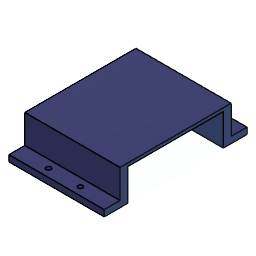
CubrePilas (Autodesk Fusion 360 design; units mm, degrees)
Autodesk Fusion 360 part; units mm, degrees
note: some values were not read from the file. Set by a fixed rule: which sketch regions a step uses.
sketch "Boceto2" plane through (0, 4, 0) normal (0, 1, 0) x (-1, 0, 0)
  line L0 (9, 0) -> (-1, 0)
  line L1 (-30, 0) -> (-60, 0)
  line L2 (-30, 0) -> (0, 0)
  line L3 (-30, 25) -> (-30, -10)
  line L4 (-30, -10) -> (-60, -10)
  line L5 (-60, -10) -> (-60, 60)
  line L6 (-60, 60) -> (0, 60)
  line L7 (0, 60) -> (0, -10)
  line L8 (0, -10) -> (-30, -10)
  line L9 (0, -10) -> (-5, -10)
  line L10 (-5, -10) -> (-5, -5)
  line L11 (-5, -5) -> (-55, -5)
  line L12 (-55, -5) -> (-55, 55)
  line L13 (-55, 55) -> (-5, 55)
  line L14 (-5, 55) -> (-5, -5)
  dimension "d1" = 10
  dimension "d2" = 30
  dimension "d3" = 30
  dimension "d4" = 35
  dimension "d5" = 70
  dimension "d6" = 5
  dimension "d7" = 5
  dimension "d8" = 50
  dimension "d9" = 60
  constraint horizontal L0
  constraint horizontal L1
  constraint parallel L1 L2
  constraint perpendicular L2 L3
  constraint perpendicular L3 L4
  constraint perpendicular L1 L5
  constraint perpendicular L3 L6
  constraint perpendicular L4 L7
  constraint perpendicular L3 L8
  constraint perpendicular L7 L9
  constraint perpendicular L9 L10
  constraint perpendicular L5 L11
  constraint perpendicular L1 L12
  constraint perpendicular L12 L13
  constraint perpendicular L11 L14
  measures "d1" distance of L0.start L0.end
  measures "d2" distance of L1.start L1.end
  measures "d3" distance of L1.start L2.end
  measures "d4" distance of L3.start L3.end
  measures "d5" distance of L4.end L5.end
  measures "d6" distance of L7.end L9.end
  measures "d7" distance of L9.end L10.end
  measures "d8" distance of L10.end L11.end
  measures "d9" distance of L11.end L12.end
extrude "Extruir1" add sketch "Boceto2" along normal blind 20 contours L0 L2 L7 L8 L9 L10 L14 | L0 L1 L2 L5 L6 L7 L12 L13 L14 | L3 L8 L10 L11 | L1 L3 L4 L5 L11 L12
sketch "Boceto3" plane through (0, 4, 0) normal (0, 1, 0) x (-1, 0, 0)
  line L0 (0, -10) -> (-5, -10)
  line L1 (-5, -10) -> (-10, -20)
  line L2 (0, -10) -> (0, -20)
  line L3 (0, -20) -> (-60, -20)
  line L4 (-60, -20) -> (-60, -10)
  line L5 (-60, -10) -> (-64.5056, 6.5239)
  line L6 (0, 60) -> (0, 70)
  line L7 (0, 70) -> (-60, 70)
  line L8 (-60, 70) -> (-60, 60)
  line L9 (-60, 60) -> (0, 60)
  line L10 (-5, -10) -> (-60, -10)
  dimension "d12" = 10
  dimension "d13" = 10
  constraint horizontal L0
  constraint perpendicular L0 L2
  constraint perpendicular L2 L3
  constraint perpendicular L3 L4
  constraint vertical L6
  constraint perpendicular L6 L7
  constraint perpendicular L7 L8
  constraint perpendicular L6 L9
  constraint perpendicular L4 L10
  measures "d12" distance of L0.start L2.end
  measures "d13" distance of L6.start L6.end
extrude "Extruir2" add sketch "Boceto3" along normal blind 4
sketch "Boceto4" plane through (0, 8, 0) normal (0, 1, 0) x (-1, 0, 0)
  line L0 (0, -10) -> (-60, -10)
  line L1 (-60, -10) -> (-60, -20)
  line L2 (-60, -20) -> (0, -20)
  line L3 (0, -20) -> (0, -10)
  line L4 (0, -15) -> (-20, -15)
  line L5 (-26, -15) -> (-35, -15)
  line L6 (-20, -15) -> (-40, -15)
  line L7 (-40, -15) -> (-80, 70)
  line L8 (0, 70) -> (0, 65)
  line L9 (0, 65) -> (-20, 65)
  line L10 (-20, 65) -> (-40, 65)
  circle A0 centre (-40, 65) radius 1.5
  circle A1 centre (-20, 65) radius 1.5
  circle A2 centre (-20, -15) radius 1.5
  circle A3 centre (-40, -15) radius 1.5
  dimension "d16" = 20
  dimension "d17" = 3
  dimension "d18" = 3
  dimension "d19" = 3
  dimension "d20" = 3
  constraint midpoint L3 L4.start
  constraint perpendicular L1 L4
  constraint parallel L4 L5
  constraint parallel L5 L6
  constraint vertical L8
  constraint perpendicular L8 L9
  constraint perpendicular L8 L10
  constraint coincident L10.end A0.centre
  constraint coincident L9.end L10.start
  constraint coincident L4.end L6.start
  constraint coincident L6.end L7.start
  measures "d16" distance of L4.start L4.end
  measures "d17" diameter of A0
  measures "d18" diameter of A1
  measures "d19" diameter of A2
  measures "d20" diameter of A3
extrude "Extruir3" cut sketch "Boceto4" against normal blind 30 contours L6 L7 A3 | L6 L7 A3 | L4 L6 A2 | L4 L6 A2 | L9 L10 A1 | L9 L10 A1 | A0
sketch "Boceto5" plane through (0, 24, 0) normal (0, 1, 0) x (-1, 0, 0)
  line L0 (-55, 55) -> (-5, 55)
  line L1 (-5, 55) -> (-5, -5)
  line L2 (-5, -5) -> (-55, -5)
  line L3 (-55, -5) -> (-55, 55)
  line L4 (0, -10) -> (0, 60)
  line L5 (0, 60) -> (-60, 60)
  line L6 (-60, 60) -> (-60, -10)
  line L7 (-60, -10) -> (0, -10)
  line L8 (0, -10) -> (-60, -10)
  line L9 (-60, 60) -> (-60, -10)
  line L10 (-60, 60) -> (0, 60)
  line L11 (0, -8.1337) -> (20, 20)
  line L12 (0, -10) -> (0, 60)
  constraint coincident L4.start L7.end
  constraint coincident L6.end L7.start
  constraint coincident L5.end L6.start
  constraint coincident L4.end L5.start
  constraint coincident L4 L11.start
extrude "Extruir4" add sketch "Boceto5" along normal blind 2 contours L0 L1 L2 L3 | L4 L5 L6 L7 L8 L9 L10 L12
sketch "Boceto6" plane through (60, 0, 0) normal (1, 0, 0) x (0, 0, -1)
  line L0 (-70, 4) -> (20, 4)
  line L1 (20, 4) -> (20, 8)
  line L2 (20, 8) -> (10, 8)
  line L3 (10, 8) -> (10, 26)
  line L4 (10, 26) -> (-60, 26)
  line L5 (-60, 26) -> (-60, 8)
  line L6 (-60, 8) -> (-70, 8)
  line L7 (-70, 8) -> (-70, 4)
sketch "Boceto7" plane through (0, 4, 0) normal (0, -1, 0) x (1, 0, 0)
  circle A0 centre (40, -15) radius 1.5
  circle A1 centre (20, 65) radius 1.5
  circle A2 centre (20, -15) radius 1.5
  circle A3 centre (40, 65) radius 1.5
  line L0 (5, 55) -> (55, 55)
  line L1 (55, 55) -> (55, -5)
  line L2 (55, -5) -> (5, -5)
  line L3 (5, -5) -> (5, 55)
  line L4 (0, 70) -> (0, -20)
  line L5 (0, -20) -> (60, -20)
  line L6 (60, -20) -> (60, 70)
  line L7 (60, 70) -> (0, 70)
  line L8 (5, 55) -> (0, 55)
  line L9 (5, -5) -> (0, -5)
  line L10 (0, 55) -> (0, -5)
  line L11 (5, 55) -> (5, -5)
  line L12 (55, 55) -> (60, 55)
  line L13 (60, 55) -> (60, -5)
  line L14 (55, -5) -> (60, -5)
  line L15 (55, -5) -> (55, 55)
  constraint coincident L0.start L3.end
  constraint coincident L4 L8.end
  constraint perpendicular L4 L8
  constraint coincident L2.end L3.start
  constraint coincident L4 L9.end
  constraint perpendicular L4 L9
  constraint coincident L0.end L1.start
  constraint coincident L6 L12.end
  constraint perpendicular L1 L12
  constraint coincident L6 L13.end
  constraint coincident L1.end L2.start
  constraint perpendicular L6 L14
extrude "Extruir5" cut sketch "Boceto7" against normal blind 20 contours L3 L4 L8 L9 L10 L11 | L1 L6 L12 L13 L14 L15
